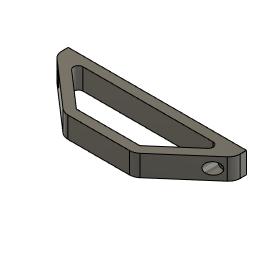
sensoree_1.0 (Autodesk Fusion 360 design; units mm, degrees)
Autodesk Fusion 360 part; units mm, degrees
sketch "Sketch1" plane through (0, 0, 0) normal (0, 1, 0) x (1, 0, 0)
  line L0 (0, 0) -> (-33, 0)
  line L1 (0, 0) -> (33, 0)
  line L2 (-33, 0) -> (-38, 0)
  line L3 (33, 0) -> (38, 0)
  line L4 (-38, 0) -> (-38, -2.7218)
  line L5 (-36.2809, -6.4949) -> (-16.411, -23.773)
  line L6 (-13.1301, -25) -> (13.1301, -25)
  line L7 (38, 0) -> (38, -2.7218)
  line L8 (36.2809, -6.4949) -> (16.411, -23.773)
  arc A0 (-38, -2.7218) -> (-36.2809, -6.4949) centre (-33, -2.7218) ccw
  arc A1 (36.2809, -6.4949) -> (38, -2.7218) centre (33, -2.7218) ccw
  arc A2 (13.1301, -25) -> (16.411, -23.773) centre (13.1301, -20) ccw
  arc A3 (-16.411, -23.773) -> (-13.1301, -25) centre (-13.1301, -20) ccw
  line L9 (0, -4) -> (27.7062, -4)
  line L10 (33, -4) -> (33.0541, -4)
  line L11 (29.0185, -7.5092) -> (13.7863, -20.7546)
  arc A4 (13.1301, -21) -> (13.7863, -20.7546) centre (13.1301, -20) ccw
  line L12 (-13.1301, -21) -> (13.1301, -21)
  arc A5 (-13.7863, -20.7546) -> (-13.1301, -21) centre (-13.1301, -20) ccw
  line L13 (-29.0185, -7.5092) -> (-13.7863, -20.7546)
  line L14 (-33, -4) -> (-33.0541, -4)
  line L15 (0, -4) -> (-27.7062, -4)
  arc A6 (-27.7062, -4) -> (-29.0185, -7.5092) centre (-27.7062, -6) ccw
  arc A7 (29.0185, -7.5092) -> (27.7062, -4) centre (27.7062, -6) ccw
  dimension "d2" = 5
  dimension "d3" = 2
  dimension "d4" = 2
  constraint coincident L0.start L1.start
  constraint horizontal L0
  constraint parallel L0 L1
  constraint parallel L0 L2
  constraint parallel L1 L3
  constraint perpendicular L2 L4
  constraint perpendicular L4 L6
  constraint perpendicular L3 L7
  constraint tangent L4 A0
  constraint tangent L5 A0
  constraint tangent L7 A1
  constraint tangent L8 A1
  constraint equal A0 A1
  constraint tangent L6 A2
  constraint tangent L8 A2
  constraint equal A0 A2
  constraint tangent L5 A3
  constraint tangent L6 A3
  constraint equal A0 A3
  constraint parallel L1 L9
  constraint parallel L3 L10
  constraint parallel L8 L11
  constraint concentric A2 A4
  constraint parallel L6 L12
  constraint concentric A3 A5
  constraint parallel L5 L13
  constraint parallel L2 L14
  constraint parallel L0 L15
  constraint tangent L12 A5
  constraint tangent A4 L12
  constraint tangent L11 A4
  constraint tangent A5 L13
  constraint coincident L14.start L15
  constraint coincident L14.end L13
  constraint tangent L15 A6
  constraint tangent L13 A6
  constraint coincident L10.end L11
  constraint coincident L10.start L9
  constraint tangent L11 A7
  constraint tangent L9 A7
  measures "d2" radius of A0
  measures "d3" radius of A6
  measures "d4" radius of A7
extrude "Extrude1" add sketch "Sketch1" along normal blind 9
sketch "Sketch2" plane through (0, 0, 0) normal (0, 0, -1) x (-1, 0, 0)
  line L0 (-38, 0) -> (38, 0)
  line L1 (38, 0) -> (38, 9)
  line L2 (38, 9) -> (-38, 9)
  line L3 (-38, 9) -> (-38, 0)
  line L4 (0, 0) -> (0, 9)
  line L5 (0, 4.5) -> (-33, 4.5)
  line L6 (0, 4.5) -> (33, 4.5)
  dimension "d7" = 33
  dimension "d8" = 33
  constraint coincident L4.start origin
  constraint midpoint L2 L4.end
  constraint midpoint L4 L5.start
  constraint perpendicular L4 L5
  constraint perpendicular L4 L6
  measures "d7" distance of L5.start L5.end
  measures "d8" distance of L5.start L6.end
hole "Hole1" at (33, 4.5, 0) at (-33, 4.5, 0) direction (0, 0, 1) diameter 3 depth 122 tip angle 180
sketch "Sketch3" plane through (0, 0, 25) normal (0, 0, 1) x (1, 0, 0)
  line L0 (-13.1301, 0) -> (13.1301, 0)
  line L1 (13.1301, 0) -> (13.1301, 9)
  line L2 (13.1301, 9) -> (-13.1301, 9)
  line L3 (-13.1301, 9) -> (-13.1301, 0)
  line L4 (0, 0) -> (0, 9)
  line L5 (0, 4.5) -> (-33, 4.5)
  line L6 (0, 4.5) -> (33, 4.5)
  dimension "d12" = 33
  dimension "d13" = 33
  constraint coincident L4.start origin
  constraint midpoint L2 L4.end
  constraint midpoint L4 L5.start
  constraint perpendicular L4 L5
  constraint perpendicular L4 L6
  measures "d12" distance of L5.start L5.end
  measures "d13" distance of L5.start L6.end
hole "Hole2" at (33, 4.5, 25) at (-33, 4.5, 25) direction (0, 0, -1) diameter 5 depth 20 tip angle 180
